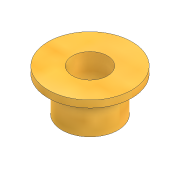
# Autodesk Inventor part: Buje para Tornillo
Saved by Autodesk Inventor 2020.3 (Build 243373000, 373)
## iProperties
Created: 2020-05-11
Part Number: Buje para Tornillo
Material: Brass, Soft Yellow
Document SubType Name: Modeling
Designer: Dante
Density: 8.47 g/cm^3
Appearance: Bamboo
Mass: 1.28177 g
Surface Area: 14.8283 cm^2
Volume: 1.28177 cm^3
Author: Dante
Autodesk Inventor part; units mm, degrees
ref_plane "YZ Plane" through (0, 0, 0) normal (1, 0, 0) x (0, 1, 0)
ref_plane "XZ Plane" through (0, 0, 0) normal (0, 1, 0) x (-1, 0, 0)
ref_plane "XY Plane" through (0, 0, 0) normal (0, 0, 1) x (1, 0, 0)
sketch "Sketch1" plane through (0, 0, 0) normal (0, 0, 1) x (1, 0, 0)
  line L0 (-11, 0) -> (-14, 0)
  line L1 (-14, 0) -> (-14, 10)
  line L2 (-14, 10) -> (-18, 10)
  line L3 (-18, 10) -> (-18, 12)
  line L4 (-18, 12) -> (-11, 12)
  line L5 (-11, 10) -> (-11, 0)
  line L6 (-11, 10) -> (-11, 12)
  line L7 (-6, 0) -> (-6, 10)
  dimension "d1" = 10
  dimension "d2" = 4
  dimension "d3" = 2
  dimension "d4" = 3
  dimension "d6" = 5
  constraints: 16 end point, 5 perpendicular, 2 vertical, 1 horizontal
  measures "d1" distance of L0.end L1.end
  measures "d2" distance of L1.end L2.end
  measures "d3" distance of L2.end L3.end
  measures "d4" distance between parallel lines of L1 L5
  measures "d6" distance between parallel lines of L7 L5
revolve "Revolution1" add sketch "Sketch1" angle 360 about axis through (-6, 0, 0) along (0, 1, 0)
body "Solid1"
